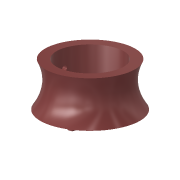
# Autodesk Inventor part: geneva_tension
Saved by Autodesk Inventor 2018 (Build 220112000, 112)
## iProperties
Created: 2018-11-13
Part Number: geneva_tension
Material: Generic
Document SubType Name: Modeling
Designer: Koki
Density: 1 g/cm^3
Appearance: Chestnut
Author: Koki
Autodesk Inventor part; units mm, degrees
note: some values were not read from the file. Chosen so that the rebuilt part matches the saved one: edges of "Fillet2".
ref_plane "YZ Plane" through (0, 0, 0) normal (1, 0, 0) x (0, 1, 0)
ref_plane "XZ Plane" through (0, 0, 0) normal (0, 1, 0) x (-1, 0, 0)
sketch "Sketch1" plane through (0, 0, 0) normal (0, 1, 0) x (-1, 0, 0)
  circle A0 centre (0, 0) radius 10.3057
  dimension "d0" = 20.6114
  constraints: 1 centre point, 1 coincident
  measures "d0" diameter of A0
extrude "Extrusion1" add sketch "Sketch1" along normal blind 4
sketch "Sketch2" plane through (0, 4, 0) normal (0, 1, 0) x (1, 0, 0)
  line L0 (0, 0) -> (0, 20.6114)
  circle A0 centre (0, 20.6114) radius 14.85
  dimension "d3" = 20.6114
  dimension "d4" = 29.7
  constraints: 2 end point, 1 centre point, 1 coincident, 1 vertical
  measures "d3" distance of L0.start L0.end
  measures "d4" diameter of A0
extrude "Extrusion2" cut sketch "Sketch2" against normal blind 4
pattern_circular "Circular Pattern1" count 3 over 360 about axis through (0, -10, 0) along (0, 1, 0) of "Extrusion2"
sketch "Sketch3" plane through (0, 4, 0) normal (0, 1, 0) x (1, 0, 0)
  line L0 (1.25, -10.3057) -> (-1.25, -10.3057)
  line L1 (-1.25, -10.3057) -> (-1.25, -2.7614)
  line L2 (-1.25, -2.7614) -> (1.25, -2.7614)
  line L3 (1.25, -2.7614) -> (1.25, -10.3057)
  arc A0 (-3.0068, -9.8573) -> (3.0068, -9.8573) centre (0, 0) ccw projected
  arc A1 (1.25, -2.7614) -> (-1.25, -2.7614) centre (0, -2.7614) ccw
  point P0 (0, -10.3057)
  dimension "d10" = 2.5
  dimension "d11" = 1.25
  dimension "d12" = 7.5443
  constraints: 8 end point, 3 point on circle, 2 midpoint, 2 parallel, 1 centre point, 1 horizontal, 1 perpendicular
  measures "d10" distance of L0.start L0.end
  measures "d11" distance from line of point (0, 0) L3
  measures "d12" distance of L2.end L0.start
extrude "Extrusion3" cut sketch "Sketch3" against normal blind 4
pattern_circular "Circular Pattern2" count 3 over 360 about axis through (0, -10, 0) along (0, 1, 0) of "Extrusion3"
sketch "Sketch4" plane through (0, 4, 0) normal (0, 1, 0) x (1, 0, 0)
  circle A0 centre (0, 0) radius 1.15
  dimension "d18" = 2.3
  constraints: 1 centre point, 1 coincident
  measures "d18" diameter of A0
extrude "Extrusion4" cut sketch "Sketch4" against normal through all
sketch "Sketch5" plane through (0, 4, 0) normal (0, 1, 0) x (1, 0, 0)
  circle A0 centre (0, 0) radius 2.625
  circle A1 centre (0, 0) radius 3.625
  dimension "d21" = 5.25
  dimension "d22" = 7.25
  constraints: 2 centre point, 2 coincident
  measures "d21" diameter of A0
  measures "d22" diameter of A1
extrude "Extrusion5" add sketch "Sketch5" along normal blind 2.9
sketch "Sketch6" plane through (0, 4, 0) normal (0, 1, 0) x (1, 0, 0)
  circle A0 centre (0, 0) radius 2.625 projected
extrude "Extrusion6" add sketch "Sketch6" along normal blind 0.4
ref_plane "Work Plane3" through (0, 24, 0) normal (0, 1, 0) x (1, 0, 0)
ref_plane "Work Plane2" through (0, 14, 0) normal (0, 1, 0) x (1, 0, 0)
sketch "Sketch7" plane through (0, 4, 0) normal (0, 1, 0) x (1, 0, 0)
  circle A0 centre (0, 0) radius 18.5
  dimension "d30" = 37
  constraints: 1 centre point, 1 coincident
  measures "d30" diameter of A0
sketch "Sketch8" plane through (0, 14, 0) normal (0, 1, 0) x (1, 0, 0)
  circle A0 centre (0, 0) radius 15
  dimension "d31" = 30
  constraints: 1 centre point, 1 coincident
  measures "d31" diameter of A0
sketch "Sketch9" plane through (0, 24, 0) normal (0, 1, 0) x (1, 0, 0)
  circle A0 centre (0, 0) radius 18.5
  dimension "d32" = 37
  constraints: 1 centre point, 1 coincident
  measures "d32" diameter of A0
loft "Loft1" add profiles "Sketch7", "Sketch8", "Sketch9"
sketch "Sketch10" plane through (0, 24, 0) normal (0, 1, 0) x (1, 0, 0)
  circle A0 centre (0, 0) radius 6
  dimension "d39" = 12
  constraints: 1 centre point, 1 coincident
  measures "d39" diameter of A0
extrude "Extrusion7" cut sketch "Sketch10" against normal blind 20
sketch "Sketch11" plane through (0, 4, 0) normal (0, 1, 0) x (1, 0, 0)
  circle A0 centre (0, 0) radius 2.675
  circle A1 centre (0, 0) radius 3.625
  dimension "d42" = 5.35
  dimension "d43" = 7.25
  constraints: 2 centre point, 2 coincident
  measures "d42" diameter of A0
  measures "d43" diameter of A1
extrude "Extrusion8" add sketch "Sketch11" along normal blind 2.9
sketch "Sketch12" plane through (0, 4, 0) normal (0, 1, 0) x (1, 0, 0)
  circle A0 centre (0, 0) radius 2.675 projected
extrude "Extrusion9" add sketch "Sketch12" along normal blind 0.4
sketch "Sketch13" plane through (0, 0, 0) normal (0, -1, 0) x (1, 0, 0)
  circle A0 centre (0, 0) radius 1.15 projected
extrude "Extrusion10" cut sketch "Sketch13" along normal through all both and the other way through all
fillet "Fillet2" radius 1 3 edges at (0, 4, -3.625) (-3.1393, 4, 1.8125) (3.6117, 4, -0.3105)
fillet "Fillet3" [suppressed]
sketch "Sketch14" plane through (0, 0, 0) normal (1, 0, 0) x (0, 1, 0)
  circle A0 centre (14, 0) radius 1
  line L0 (0, -2.3247) -> (0, 9.8573) projected
  point P0 (0, 0)
  dimension "d53" = 2
  dimension "d54" = 14
  constraints: 1 centre point
  measures "d53" diameter of A0
  measures "d54" distance from line of L0 A0.centre
extrude "Extrusion11" cut sketch "Sketch14" against normal through all
sketch "Sketch15" plane through (0, 24, 0) normal (0, 1, 0) x (1, 0, 0)
  circle A0 centre (0, 0) radius 12.5
  dimension "d57" = 25
  constraints: 1 centre point, 1 coincident
  measures "d57" diameter of A0
extrude "Extrusion13" cut sketch "Sketch15" against normal blind 15
fillet "Fillet4" [suppressed]
sketch "Sketch16" plane through (0, 0, 0) normal (1, 0, 0) x (0, 1, 0)
  line L0 (29.1935, -29.1286) -> (21, -29.1286)
  line L1 (21, -29.1286) -> (21, 23.6081)
  line L2 (21, 23.6081) -> (29.1935, 23.6081)
  line L3 (29.1935, 23.6081) -> (29.1935, -29.1286)
  line L4 (24, 18.5) -> (24, -18.5) projected
  point P0 (0, 0)
  point P1 (24, 0)
  dimension "d64" = 3
  constraints: 8 end point, 2 parallel, 1 horizontal, 1 perpendicular
  measures "d64" distance between parallel lines of L1 L4
extrude "Extrusion14" cut sketch "Sketch16" along normal through all both and the other way through all
sketch "Sketch17" plane through (0, 6.9, 0) normal (0, 1, 0) x (1, 0, 0)
  circle A0 centre (0, 0) radius 3.625 projected
  circle A1 centre (0, 0) radius 2.675 projected
extrude "Extrusion15" add sketch "Sketch17" along normal blind 3.5
sketch "Sketch18" plane through (0, 4.4, 0) normal (0, 1, 0) x (1, 0, 0)
  circle A0 centre (0, 0) radius 1.15 projected
  circle A1 centre (0, 0) radius 1.15 projected
  circle A2 centre (0, 0) radius 2.675 projected
extrude "Extrusion16" add sketch "Sketch18" along normal blind 3.5
sketch "Sketch19" plane through (-0.0069, 21, 0.0099) normal (0, 1, 0) x (1, 0, 0)
  circle A0 centre (0.0069, 0.0099) radius 16.715
  dimension "d71" = 33.43
  constraints: 1 centre point, 1 coincident, 1 other
  measures "d71" diameter of A0
ref_plane "Work Plane1" through (0, 4, 0) normal (0, 1, 0) x (1, 0, 0)
equation "\"d11\" = 0.5 * d10"
body "Solid1"
